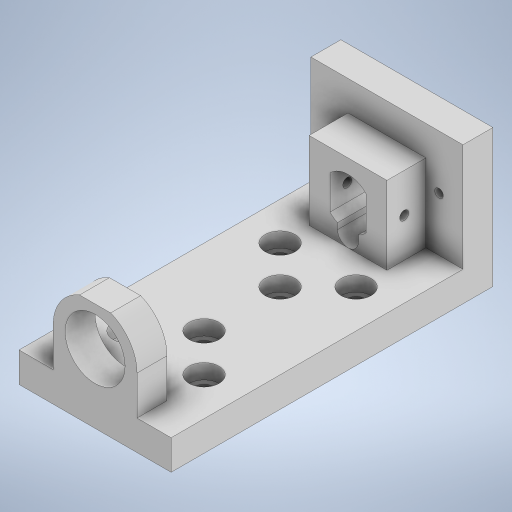
# Autodesk Inventor part: Actuator Stage Actuator Mount V0.2
Saved by Autodesk Inventor 2024 (Build 280153000, 153)
## iProperties
Created: 2024-10-02
Part Number: Actuator Stage Actuator Mount V0.2
Material: Generic
Document SubType Name: Modeling
Designer: Scott
Density: 1 g/cm^3
Appearance: Default
Author: Scott
Autodesk Inventor part; units mm, degrees
ref_plane "YZ Plane" through (0, 0, 0) normal (1, 0, 0) x (0, 1, 0)
ref_plane "XZ Plane" through (0, 0, 0) normal (0, 1, 0) x (-1, 0, 0)
sketch "Sketch1" plane through (0, 0, 0) normal (0, 0, 1) x (1, 0, 0)
  line L0 (-22.1831, 0) -> (-47.5831, 0)
  line L1 (0, 0) -> (50.8, 0)
  line L2 (50.8, 0) -> (50.8, 5)
  line L3 (50.8, 5) -> (50.8, 10)
  line L4 (50.8, 10) -> (50.8, 36)
  line L5 (50.8, 36) -> (50.8, 46)
  line L6 (50.8, 46) -> (0, 46)
  line L7 (0, 46) -> (0, 0)
  dimension "d0" = 25.4
  dimension "d1" = 50.8
  dimension "d2" = 5
  dimension "d3" = 5
  dimension "d4" = 26
  dimension "d5" = 10
  constraints: 16 end point, 3 point on line, 2 horizontal, 2 perpendicular, 1 vertical
  measures "d0" distance of L0.start L0.end
  measures "d1" distance of L1.start L1.end
  measures "d2" distance of L1.end L2.end
  measures "d3" distance of L2.end L3.end
  measures "d4" distance of L3.end L4.end
  measures "d5" distance of L4.end L5.end
extrude "Extrusion1" add sketch "Sketch1" along normal blind 10
sketch "Sketch2" plane through (0, 0, 10) normal (0, 0, 1) x (1, 0, 0)
  line L0 (50.8, 0) -> (50.8, 46) projected
  line L1 (50.8, 46) -> (0, 46) projected
  line L2 (0, 46) -> (0, 0) projected
  line L3 (0, 0) -> (50.8, 0) projected
  line L4 (0, 46) -> (0, 0) projected
  line L5 (0, 0) -> (50.8, 0)
  line L6 (50.8, 0) -> (50.8, 46) projected
  line L7 (50.8, 0) -> (50.8, 10)
  line L8 (50.8, 10) -> (0, 10)
  line L9 (0, 0) -> (0, 10)
  dimension "d8" = 10
  constraints: 8 end point, 3 perpendicular, 2 point on line
  measures "d8" distance of L0.start L7.end
extrude "Extrusion2" add sketch "Sketch2" along normal blind 87.5 contours L3 L2 L8 L0
sketch "Sketch3" plane through (0, 0, 10) normal (0, 0, 1) x (1, 0, 0)
  line L0 (0, 10) -> (50.8, 10) projected
  line L1 (50.8, 10) -> (50.8, 46) projected
  line L2 (50.8, 46) -> (0, 46) projected
  line L3 (0, 46) -> (0, 10) projected
  line L4 (12.4, 36) -> (38.4, 36)
  line L5 (38.4, 36) -> (38.4, 10)
  line L6 (38.4, 10) -> (12.4, 10)
  line L7 (12.4, 10) -> (12.4, 36)
  line L8 (17.4, 31) -> (33.4, 31)
  line L9 (33.4, 31) -> (33.4, 15)
  line L10 (33.4, 15) -> (17.4, 15)
  line L11 (17.4, 15) -> (17.4, 31)
  point P0 (0, 0)
  dimension "d1" = 50.8
  dimension "d12" = 38.4
  dimension "d13" = 10
  dimension "d14" = 5
  dimension "d15" = 5
  dimension "d16" = 16
  dimension "d17" = 16
  dimension "d18" = 5
  dimension "d19" = 5
  dimension "d24" = 26
  dimension "d26" = 26
  constraints: 16 end point, 4 parallel, 2 horizontal, 2 perpendicular
  measures "d12" distance between parallel lines of L3 L5
  measures "d13" distance between parallel lines of L2 L4
  measures "d14" distance between parallel lines of L4 L8
  measures "d15" distance between parallel lines of L6 L10
  measures "d16" distance between parallel lines of L8 L10
  measures "d17" distance between parallel lines of L11 L9
  measures "d18" distance between parallel lines of L5 L9
  measures "d19" distance between parallel lines of L7 L11
  measures "d24" distance of L6.end L4.start
  measures "d26" distance of L5.end L6.end
extrude "Extrusion3" add sketch "Sketch3" along normal blind 13 contours L7 L4 L5 L0 | L8 L9 L10 L11
sketch "Sketch5" plane through (0, 0, 0) normal (0, 0, -1) x (-1, 0, 0)
  line L0 (-12.4, 36) -> (-38.4, 36) projected
  line L1 (-38.4, 36) -> (-38.4, 10) projected
  line L2 (-12.4, 10) -> (-12.4, 36) projected
  line L3 (0, 10) -> (-12.4, 10) projected
  line L4 (-50.8, 10) -> (-50.8, 46) projected
  line L5 (-50.8, 46) -> (0, 46) projected
  line L6 (0, 46) -> (0, 10) projected
  line L7 (0, 0) -> (-50.8, 0) projected
  line L8 (-50.8, 0) -> (-50.8, 10) projected
  line L9 (-50.8, 10) -> (0, 10) projected
  line L10 (0, 10) -> (0, 0) projected
  circle A0 centre (-42.8, 28) radius 1.42
  circle A1 centre (-8, 28) radius 1.42
  line L11 (-38.4, 10) -> (-50.8, 10) projected
  dimension "d29" = 2.84
  dimension "d30" = 2.84
  dimension "d31" = 8
  dimension "d32" = 8
  dimension "d33" = 8
  dimension "d34" = 8
  constraints: 2 centre point
  measures "d29" diameter of A0
  measures "d30" diameter of A1
  measures "d31" distance from line of L4 A0.centre
  measures "d32" distance from line of L6 A1.centre
  measures "d33" distance from line of L0 A1.centre
  measures "d34" distance from line of L0 A0.centre
extrude "Extrusion5" cut sketch "Sketch5" against normal blind 26 contours A0 | A1
sketch "Sketch9" plane through (0, 0, 0) normal (0, 0, -1) x (-1, 0, 0)
  circle A0 centre (-8, 28) radius 1.42 projected
  circle A1 centre (-42.8, 28) radius 1.42 projected
  line L0 (-50.8, 0) -> (-50.8, 46) projected
  line L1 (0, 0) -> (-50.8, 0) projected
  line L2 (0, 46) -> (0, 0) projected
  line L3 (-50.8, 46) -> (0, 46) projected
  circle A2 centre (-42.8, 28) radius 1.42 projected
  circle A3 centre (-42.8, 28) radius 5
  circle A4 centre (-8, 28) radius 1.42 projected
  circle A5 centre (-8, 28) radius 5
  dimension "d55" = 10
  dimension "d56" = 10
  constraints: 2 centre point, 2 coincident
  measures "d55" diameter of A3
  measures "d56" diameter of A5
extrude "Extrusion9" cut sketch "Sketch9" against normal blind 5 contours A3 | A5
sketch "Sketch7" plane through (0, 0, 23) normal (0, 0, 1) x (1, 0, 0)
  line L0 (12.4, 36) -> (12.4, 10) projected
  line L1 (38.4, 10) -> (38.4, 36) projected
  line L2 (38.4, 36) -> (12.4, 36) projected
  circle A0 centre (25.4, 23) radius 8.25
  circle A1 centre (25.4, 23) radius 6
  line L3 (19.4, 28.6624) -> (19.4, 17.3376)
  line L4 (38.4, 10) -> (12.4, 10) projected
  line L5 (31.4, 28.6624) -> (31.4, 17.3376)
  point P0 (0, 0)
  dimension "d42" = 26
  dimension "d43" = 16.5
  dimension "d45" = 13
  dimension "d46" = 12
  dimension "d59" = 26
  dimension "d61" = 0
  dimension "d62" = 180
  dimension "d69" = 0
  dimension "d99" = 13
  constraints: 4 end point, 4 point on circle, 2 centre point, 1 coincident, 1 vertical
  measures "d42" distance of L1.end L0.start
  measures "d43" diameter of A0
  measures "d45" distance from line of L0 A0.centre
  measures "d46" diameter of A1
  measures "d59" distance of L0.start L0.end
  measures "d61" distance edge to line of A1 L3
  measures "d62" angle of L0 L3
  measures "d69" distance edge to line of A1 L5
  measures "d99" distance from line of L2 A0.centre
extrude "Extrusion7" cut sketch "Sketch7" against normal blind 14 contours L5 A1 L3 A0 | A0 L3 A1 L5 | A1
sketch "Sketch10" plane through (38.4, 10, 10) normal (1, 0, 0) x (0, 0, -1)
  line L0 (-13, 7.3376) -> (-13, 18.6624) projected
  line L1 (-13, 7.3376) -> (1, 7.3376) projected
  line L2 (1, 7.3376) -> (1, 18.6624) projected
  line L3 (-13, 18.6624) -> (1, 18.6624) projected
  circle A0 centre (-7.25, 13) radius 1.5
  point P0 (10, -10)
  dimension "d63" = 3
  dimension "d64" = 8.25
  dimension "d65" = 11.3247
  dimension "d66" = 5.6624
  constraints: 1 centre point
  measures "d63" diameter of A0
  measures "d64" distance from line of L2 A0.centre
  measures "d65" distance of L0.start L0.end
  measures "d66" distance from line of L1 A0.centre
extrude "Extrusion10" cut sketch "Sketch10" against normal through all contours A0
sketch "Sketch11" plane through (0, 10, 97.5) normal (0, 1, 0) x (1, 0, 0)
  line L0 (38.4, 87.5) -> (38.4, 74.5) projected
  line L1 (38.4, 74.5) -> (12.4, 74.5) projected
  line L2 (12.4, 74.5) -> (12.4, 87.5) projected
  line L3 (0, 87.5) -> (12.4, 87.5) projected
  line L4 (0, 87.5) -> (0, 0) projected
  line L5 (50.8, 0) -> (0, 0) projected
  line L6 (50.8, 87.5) -> (50.8, 0) projected
  line L7 (38.4, 87.5) -> (50.8, 87.5) projected
  circle A0 centre (50.8, 77.2) radius 3.175
  circle A1 centre (38.1, 64.5) radius 3.175
  line L8 (38.4, 74.5) -> (12.4, 74.5) projected
  line L9 (38.4, 74.5) -> (25.4, 74.5)
  circle A2 centre (25.4, 77.2) radius 3.175
  circle A3 centre (12.7, 64.5) radius 3.175
  circle A4 centre (0, 77.2) radius 3.175
  circle A5 centre (-12.7, 64.5) radius 3.175
  circle A6 centre (-25.4, 77.2) radius 3.175
  circle A7 centre (-38.1, 64.5) radius 3.175
  circle A8 centre (50.8, 51.8) radius 3.175
  circle A9 centre (38.1, 39.1) radius 3.175
  circle A10 centre (25.4, 51.8) radius 3.175
  circle A11 centre (12.7, 39.1) radius 3.175
  circle A12 centre (0, 51.8) radius 3.175
  circle A13 centre (-12.7, 39.1) radius 3.175
  circle A14 centre (-25.4, 51.8) radius 3.175
  circle A15 centre (-38.1, 39.1) radius 3.175
  circle A16 centre (50.8, 26.4) radius 3.175
  circle A17 centre (38.1, 13.7) radius 3.175
  circle A18 centre (25.4, 26.4) radius 3.175
  circle A19 centre (12.7, 13.7) radius 3.175
  circle A20 centre (0, 26.4) radius 3.175
  circle A21 centre (-12.7, 13.7) radius 3.175
  circle A22 centre (-25.4, 26.4) radius 3.175
  circle A23 centre (-38.1, 13.7) radius 3.175
  circle A24 centre (50.8, 1) radius 3.175
  circle A25 centre (38.1, -11.7) radius 3.175
  circle A26 centre (25.4, 1) radius 3.175
  circle A27 centre (12.7, -11.7) radius 3.175
  circle A28 centre (0, 1) radius 3.175
  circle A29 centre (-12.7, -11.7) radius 3.175
  circle A30 centre (-25.4, 1) radius 3.175
  circle A31 centre (-38.1, -11.7) radius 3.175
  point P0 (0, 97.5)
  dimension "d70" = 26
  dimension "d71" = 6.35
  dimension "d72" = 6.35
  dimension "d73" = 13
  dimension "d75" = 12.7
  dimension "d76" = 12.7
  dimension "d77" = 10.3
  dimension "d78" = 13
  dimension "d82" = 25.4
  dimension "d85" = 25.4
  dimension "d88" = 12.7
  constraints: 32 centre point, 2 end point, 1 horizontal, 1 midpoint, 1 vertical, 60 other
  measures "d70" distance of L0.end L1.end
  measures "d71" diameter of A0
  measures "d72" diameter of A1
  measures "d73" distance of L0.end L9.end
  measures "d75" horizontal distance of A0.centre A1.centre
  measures "d76" horizontal distance of A0.centre A1.centre
  measures "d77" distance from line of L7 A0.centre
  measures "d78" distance of L0.start L0.end
  measures "d82" distance of A0.centre A2.centre
  measures "d85" distance of A0.centre A8.centre
  measures "d88" horizontal distance of L9.end A1.centre
extrude "Extrusion11" cut sketch "Sketch11" against normal blind 10 contours A1 | A3 | A10
sketch "Sketch12" plane through (0, 10, 97.5) normal (0, 1, 0) x (1, 0, 0)
  circle A0 centre (38.1, 64.5) radius 3.175 projected
  circle A1 centre (25.4, 51.8) radius 3.175 projected
  circle A2 centre (12.7, 64.5) radius 3.175 projected
  line L0 (38.4, 87.5) -> (38.4, 74.5) projected
  line L1 (38.4, 74.5) -> (12.4, 74.5) projected
  line L2 (12.4, 74.5) -> (12.4, 87.5) projected
  line L3 (0, 87.5) -> (12.4, 87.5) projected
  line L4 (0, 87.5) -> (0, 0) projected
  line L5 (50.8, 0) -> (0, 0) projected
  line L6 (50.8, 87.5) -> (50.8, 0) projected
  line L7 (38.4, 87.5) -> (50.8, 87.5) projected
  circle A3 centre (12.7, 64.5) radius 5
  circle A4 centre (25.4, 51.8) radius 5
  circle A5 centre (38.1, 64.5) radius 3.175 projected
  circle A6 centre (38.1, 64.5) radius 5
  point P0 (0, 97.5)
  dimension "d91" = 10
  dimension "d92" = 10
  dimension "d93" = 10
  constraints: 3 centre point, 3 coincident
  measures "d91" diameter of A3
  measures "d92" diameter of A4
  measures "d93" diameter of A6
extrude "Extrusion12" cut sketch "Sketch12" against normal blind 5 contours A0 | A1 | A2 | A3 | A4 | A6
sketch "Sketch14" plane through (0, 0, 97.5) normal (0, 0, 1) x (1, 0, 0)
  line L0 (7.7, 5) -> (17.7, 5) projected
  line L1 (50.8, 10) -> (0, 10) projected
  line L2 (0, 10) -> (0, 0) projected
  line L3 (0, 0) -> (50.8, 0) projected
  line L4 (50.8, 0) -> (50.8, 10) projected
  circle A0 centre (25.4, 23) radius 10
  circle A1 centre (25.4, 23) radius 14
  line L5 (0, 46) -> (0, 0) projected
  line L6 (0, 0) -> (50.8, 0)
  line L7 (50.8, 0) -> (50.8, 10)
  line L8 (50.8, 10) -> (0, 10)
  line L9 (0, 10) -> (0, 0)
  circle A2 centre (8, 28) radius 1.42 projected
  circle A3 centre (42.8, 28) radius 1.42 projected
  line L10 (38.4, 36) -> (38.4, 10) projected
  line L11 (38.4, 10) -> (50.8, 10) projected
  line L12 (50.8, 10) -> (50.8, 46) projected
  line L13 (50.8, 46) -> (0, 46) projected
  line L14 (0, 46) -> (0, 10) projected
  line L15 (0, 10) -> (12.4, 10) projected
  line L16 (12.4, 10) -> (12.4, 36) projected
  line L17 (12.4, 36) -> (38.4, 36) projected
  circle A4 centre (8, 28) radius 1.42 projected
  circle A5 centre (8, 28) radius 3
  circle A6 centre (42.8, 28) radius 1.42 projected
  circle A7 centre (42.8, 28) radius 3
  line L18 (11.4, 23) -> (11.4, 10)
  line L19 (39.4, 23) -> (39.4, 10)
  line L20 (33.1, 10) -> (43.1, 10) projected
  circle A8 centre (25.4, 23) radius 9
  line L21 (19.4, 17.3376) -> (19.4, 28.6624) projected
  arc A9 (19.4, 17.3376) -> (31.4, 17.3376) centre (25.4, 23) ccw projected
  line L22 (31.4, 28.6624) -> (31.4, 17.3376) projected
  arc A10 (31.4, 28.6624) -> (19.4, 28.6624) centre (25.4, 23) ccw projected
  line L23 (12.4, 36) -> (12.4, 10) projected
  line L24 (39.4, 10) -> (12.4, 10)
  line L25 (12.4, 10) -> (12.4, 36)
  line L26 (12.4, 36) -> (39.4, 36)
  line L27 (39.4, 36) -> (39.4, 10)
  point P0 (12.4, 10)
  point P1 (38.4, 28.1962)
  point P2 (30.5962, 36)
  point P3 (20.2038, 36)
  point P4 (12.4, 28.1962)
  point P5 (38.4, 17.8038)
  point P6 (12.4, 17.8038)
  dimension "d100" = 20
  dimension "d101" = 28
  dimension "d102" = 6
  dimension "d103" = 6
  dimension "d106" = 18
  dimension "d107" = 0
  dimension "d117" = 0
  constraints: 20 end point, 5 centre point, 4 coincident, 4 parallel, 3 perpendicular, 3 point on line, 2 horizontal, 2 point on circle, 1 tangent
  measures "d100" diameter of A0
  measures "d101" diameter of A1
  measures "d102" diameter of A5
  measures "d103" diameter of A7
  measures "d106" diameter of A8
  measures "d107" distance of A9.centre A0.centre
  measures "d117" distance between parallel lines of L17 L26
extrude "Extrusion14" add sketch "Sketch14" along normal blind 10 contours L4 L3 L2 L1 A1 | L1 L10 A1 L19 | L1 A1 L10 | A1 L10 | A1 L1 L16 L17 L10 | L18 A1 L16 L1 | A1 L1 | L16 A1 L1 | A1 L16
ref_plane "Work Plane1" through (0, 0, 58.4) normal (0, 0, 1) x (1, 0, 0)
mirror "Mirror1" about plane through (0, 0, 58.4) normal (0, 0, 1) of "Extrusion12", "Extrusion11"
sketch "Sketch15" plane through (0, 0, 23) normal (0, 0, 1) x (1, 0, 0)
  arc A0 (31.4, 28.6624) -> (19.4, 28.6624) centre (25.4, 23) ccw projected
  line L0 (19.4, 17.3376) -> (19.4, 28.6624) projected
  arc A1 (19.4, 17.3376) -> (31.4, 17.3376) centre (25.4, 23) ccw projected
  line L1 (31.4, 28.6624) -> (31.4, 17.3376) projected
  line L2 (19.4, 17.3376) -> (19.4, 28.6624) projected
  arc A2 (31.4, 28.6624) -> (19.4, 28.6624) centre (25.4, 23) ccw projected
  line L3 (31.4, 28.6624) -> (31.4, 17.3376) projected
  arc A3 (19.4, 17.3376) -> (31.4, 17.3376) centre (25.4, 23) ccw projected
  line L4 (12.4, 36) -> (12.4, 10) projected
  line L5 (38.4, 10) -> (12.4, 10) projected
  line L6 (38.4, 10) -> (38.4, 36) projected
  line L7 (38.4, 36) -> (12.4, 36) projected
  circle A4 centre (25.4, 13.5) radius 3.5
  line L8 (28.9, 26.8597) -> (21.9, 26.8597)
  line L9 (21.9, 11.25) -> (28.9, 11.25)
  line L10 (28.9, 11.25) -> (28.9, 19)
  line L11 (28.9, 19) -> (21.9, 19)
  line L12 (21.9, 19) -> (21.9, 11.25)
  point P0 (0, 0)
  point P1 (21.9, 13.5)
  point P2 (28.9, 13.5)
  dimension "d109" = 7
  dimension "d110" = 0
  dimension "d111" = 8.25
  dimension "d113" = 3.5
  dimension "d116" = 5.5
  constraints: 10 end point, 2 parallel, 1 centre point, 1 horizontal, 1 perpendicular
  measures "d109" diameter of A4
  measures "d110" horizontal distance of A0.centre A4.centre
  measures "d111" radius of A1
  measures "d113" distance from line of L5 A4.centre
  measures "d116" distance from line of A4.centre L11
extrude "Extrusion15" cut sketch "Sketch15" against normal through all contours L10 A4 A1 | A1 A4 L12 L11 L10 | A1 A4 L12 | A4 L9 A1 | A1 A4 | A4 L9
equation "\"d8\" = d2 + d3"
equation "\"d12\" = 0.5 * d26 + 0.5 * d1"
equation "\"d15\" = d14"
equation "\"d17\" = d16"
equation "\"d18\" = d14"
equation "\"d19\" = d14"
equation "\"d30\" = d29"
equation "\"d32\" = d31"
equation "\"d33\" = d31"
equation "\"d34\" = d31"
equation "\"d35\" = d26"
equation "\"d56\" = d55"
equation "\"d45\" = 0.5 * d42"
equation "\"d66\" = 0.5 * d65"
equation "\"d71\" = 0.25 * d0"
equation "\"d72\" = d71"
equation "\"d73\" = 0.5 * d70"
equation "\"d75\" = 0.5 * d0"
equation "\"d76\" = 0.5 * d0"
equation "\"d82\" = d0"
equation "\"d85\" = d0"
equation "\"d88\" = 0.5 * d0"
equation "\"d92\" = d91"
equation "\"d93\" = d91"
equation "\"d113\" = 0.5 * d109"
body "Solid1"
